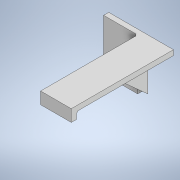
# Autodesk Inventor part: inside bracket
Saved by Autodesk Inventor 2020.3 (Build 243373000, 373)
## iProperties
Created: 2020-09-08
Part Number: inside bracket
Material: Generic
Document SubType Name: Modeling
Designer: joesp
Density: 1 g/cm^3
Appearance: Default
Author: joesp
Autodesk Inventor part; units mm, degrees
ref_plane "YZ Plane" through (0, 0, 0) normal (1, 0, 0) x (0, 1, 0)
ref_plane "XZ Plane" through (0, 0, 0) normal (0, 1, 0) x (-1, 0, 0)
ref_plane "XY Plane" through (0, 0, 0) normal (0, 0, 1) x (1, 0, 0)
sketch "Sketch1" plane through (0, 0, 0) normal (1, 0, 0) x (0, 1, 0)
  line L0 (0, 0) -> (30, 0)
  line L1 (30, 0) -> (30, 30)
  line L2 (30, 30) -> (0, 30)
  line L3 (0, 30) -> (0, 0)
  line L4 (0, 0) -> (27, 30)
  dimension "d0" = 30
  dimension "d1" = 30
  dimension "d24" = 3
  constraints: 10 end point, 2 parallel, 1 horizontal, 1 perpendicular, 1 point on line
  measures "d0" distance of L1.end L2.end
  measures "d1" distance of L0.end L1.end
  measures "d24" distance of L1.end L4.end
extrude "Extrusion1" add sketch "Sketch1" along normal blind 3 contours L4 L2 L1 L0
sketch "Sketch2" plane through (0, 0, 0) normal (-1, 0, 0) x (0, 0, 1)
  line L0 (30, 0) -> (0, 0) projected
  line L1 (0, 0) -> (3, 0)
  line L2 (3, 0) -> (3, 30)
  line L3 (3, 30) -> (0, 30)
  line L4 (0, 30) -> (0, 0)
  line L5 (0, 30) -> (30, 30) projected
  dimension "d4" = 3
  constraints: 8 end point, 2 parallel, 1 collinear, 1 horizontal, 1 perpendicular
  measures "d4" distance of L2.end L3.end
extrude "Extrusion2" add sketch "Sketch2" along normal blind 20
sketch "Sketch3" plane through (0, 0, 3) normal (0, 0, 1) x (1, 0, 0)
  circle A0 centre (-10, 14) radius 1.5
  line L0 (0, 30) -> (-20, 30) projected
  line L1 (0, 0) -> (-20, 0) projected
  line L2 (-20, 0) -> (-20, 30) projected
  line L3 (0, 30) -> (0, 0) projected
  dimension "d7" = 3
  dimension "d8" = 16
  dimension "d10" = 10
  dimension "d11" = 10
  constraints: 1 centre point
  measures "d7" diameter of A0
  measures "d8" distance from line of L0 A0.centre
  measures "d10" distance from line of L2 A0.centre
  measures "d11" distance from line of L3 A0.centre
extrude "Extrusion3" cut sketch "Sketch3" against normal through all contours A0
sketch "Sketch4" plane through (3, 0, 0) normal (1, 0, 0) x (0, 0, -1)
  line L0 (0, 0) -> (0, 30) projected
  line L1 (0, 30) -> (-60, 30)
  line L2 (-60, 30) -> (-60, 27)
  line L3 (-60, 27) -> (0, 27)
  line L4 (0, 27) -> (0, 30)
  point P0 (0, 27)
  dimension "d17" = 3
  dimension "d18" = 60
  constraints: 8 end point, 2 parallel, 1 horizontal, 1 perpendicular
  measures "d17" distance of L1.end L2.end
  measures "d18" distance of L0.end L1.end
extrude "Extrusion4" add sketch "Sketch4" along normal blind 15 and the other way blind 3
sketch "Sketch5" plane through (3, 27, 0) normal (0, -1, 0) x (1, 0, 0)
  line L0 (15, 60) -> (15, 0) projected
  line L1 (15, 60) -> (-3, 60)
  line L2 (-3, 60) -> (-3, 57)
  line L3 (-3, 57) -> (15, 57)
  line L4 (15, 57) -> (15, 60)
  line L5 (-3, 30) -> (-3, 60) projected
  point P0 (-3, 0)
  dimension "d21" = 3
  constraints: 8 end point, 2 parallel, 1 horizontal, 1 perpendicular, 1 point on line
  measures "d21" distance of L1.end L2.end
extrude "Extrusion5" add sketch "Sketch5" along normal blind 4
chamfer "Chamfer1" distance 1 angle 45 3 edges at (3, 27, 15) (0, 16.35, 3) (9, 27, 57)
equation "\"d10\" = d11"
body "Solid1"
